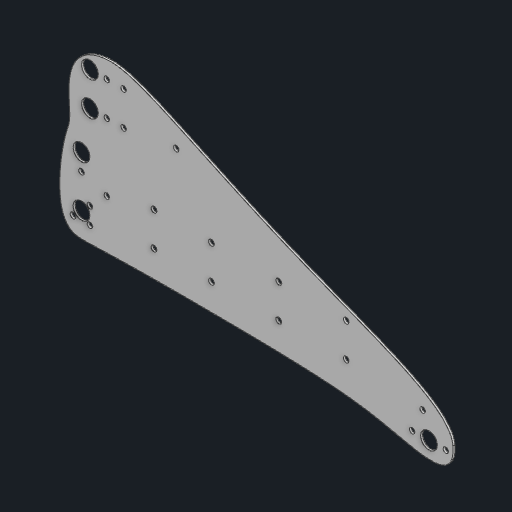
# Autodesk Inventor part: back-tower
Saved by Autodesk Inventor 2023.2 (Build 272271000, 271)
## iProperties
Created: 2023-03-28
Part Number: back-tower
Material: Generic
Document SubType Name: Modeling
Designer: eduar
Density: 1 g/cm^3
Appearance: Default
Author: eduar
Autodesk Inventor part; units mm, degrees
ref_plane "YZ Plane" through (0, 0, 0) normal (1, 0, 0) x (0, 1, 0)
ref_plane "XZ Plane" through (0, 0, 0) normal (0, 1, 0) x (-1, 0, 0)
ref_plane "XY Plane" through (0, 0, 0) normal (0, 0, 1) x (1, 0, 0)
sketch "Sketch1" plane through (0, 0, 0) normal (0, 0, 1) x (1, 0, 0)
  circle A0 centre (261.9375, -165.1) radius 6.35
  circle A1 centre (-6.35, -152.4) radius 2.1844
  circle A2 centre (0, -146.05) radius 6.35
  circle A3 centre (6.35, -139.7) radius 2.0955
  circle A4 centre (0, -120.65) radius 2.0955
  circle A5 centre (0, -107.95) radius 6.35
  circle A6 centre (31.75, -50.8) radius 2.0828
  circle A7 centre (19.05, -50.8) radius 2.0828
  circle A8 centre (31.75, -76.2) radius 2.0828
  line L0 (280.0184, -159.6357) -> (282.2244, -184.842) construction
  line L1 (282.2244, -184.842) -> (234.95, -172.2389) construction
  line L2 (234.95, -172.2389) -> (208.6659, -165.1) construction
  line L3 (208.6659, -165.1) -> (119.7894, -163.202) construction
  line L4 (119.7894, -163.202) -> (3.2359, -163.202) construction
  line L5 (3.2359, -163.202) -> (-6.35, -167.2209) construction
  line L6 (-6.35, -167.2209) -> (-20.6375, -152.4) construction
  line L7 (-20.6375, -152.4) -> (-12.7, -95.25) construction
  line L8 (-12.7, -95.25) -> (-6.35, -95.25) construction
  line L9 (-6.35, -95.25) -> (-12.7, -63.5) construction
  line L10 (-12.7, -63.5) -> (-1.5571, -41.4478) construction
  line L11 (-1.5571, -41.4478) -> (19.05, -36.5125) construction
  line L12 (19.05, -36.5125) -> (44.45, -36.5125) construction
  line L13 (44.45, -36.5125) -> (168.275, -104.775) construction
  line L14 (168.275, -104.775) -> (277.8125, -134.4295) construction
  line L15 (277.8125, -134.4295) -> (280.0184, -159.6357) construction
  spline S0 degree 4 poles (280.0184, -159.6357) (282.2244, -184.842) (234.95, -172.2389) (208.6659, -165.1) (119.7894, -163.202) (3.2359, -163.202) (-6.35, -167.2209) (-20.6375, -152.4) (-12.7, -95.25) (-6.35, -95.25) (-12.7, -63.5) (-1.5571, -41.4478) (19.05, -36.5125) (44.45, -36.5125) (168.275, -104.775) (277.8125, -134.4295) (280.0184, -159.6357) knots 0 0 0 0 0 1 2 3 4 5 6 7 8 9 10 11 12 13 13 13 13 13
  line L16 (261.9375, -165.1) -> (274.6375, -165.1)
  line L17 (261.9375, -165.1) -> (249.2375, -165.1)
  circle A9 centre (274.6375, -165.1) radius 2.0955
  circle A10 centre (249.2375, -165.1) radius 2.0955
  circle A11 centre (257.175, -147.6375) radius 2.0955
  circle A12 centre (6.35, -50.8) radius 6.35
  circle A13 centre (6.35, -76.2) radius 6.35
  circle A14 centre (19.05, -76.2) radius 2.0828
  circle A15 centre (19.05, -127) radius 2.0955
  circle A16 centre (6.35, -152.4) radius 2.0955
  circle A17 centre (71.4375, -69.85) radius 2.0955
  circle A18 centre (199.5486, -118.0725) radius 2.1971 projected
  circle A19 centre (199.5486, -143.4725) radius 2.1971 projected
  circle A20 centre (148.7486, -118.0725) radius 2.1971 projected
  circle A21 centre (148.7486, -143.4725) radius 2.1971 projected
  circle A22 centre (97.9486, -118.0725) radius 2.1971 projected
  circle A23 centre (97.9486, -143.4725) radius 2.1971 projected
  circle A24 centre (54.661, -118.0725) radius 2.1971 projected
  circle A25 centre (54.661, -143.4725) radius 2.1971 projected
  point P0 (0, 0)
  dimension "d0" = 12.7
  dimension "d1" = 12.7
  dimension "d2" = 12.7
  dimension "d3" = 4.191
  dimension "d4" = 4.191
  dimension "d7" = 4.191
  dimension "d8" = 12.7
  dimension "d9" = 4.191
  dimension "d10" = 4.191
  dimension "d11" = 4.191
  dimension "d12" = 4.191
  dimension "d13" = 12.7
  dimension "d14" = 4.1656
  dimension "d15" = 4.1656
  dimension "d16" = 4.1656
  dimension "d17" = 4.1656
  dimension "d18" = 12.7
  dimension "d19" = 12.7
  dimension "d22" = 4.191
  constraints: 18 centre point, 5 horizontal, 4 end point, 2 coincident, 2 collinear, 19 other
  measures "d0" diameter of A0
  measures "d1" distance of L16.start L16.end
  measures "d2" distance of L16.start L17.end
  measures "d3" diameter of A9
  measures "d4" diameter of A10
  measures "d7" diameter of A11
  measures "d8" diameter of A5
  measures "d9" diameter of A15
  measures "d10" diameter of A4
  measures "d11" diameter of A3
  measures "d12" diameter of A16
  measures "d13" diameter of A2
  measures "d14" diameter of A6
  measures "d15" diameter of A8
  measures "d16" diameter of A7
  measures "d17" diameter of A14
  measures "d18" diameter of A12
  measures "d19" diameter of A13
  measures "d22" diameter of A17
extrude "Extrusion3" add sketch "Sketch1" along normal blind 1.524
body "Solid3"
